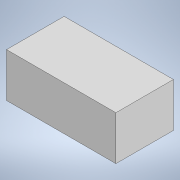
# Autodesk Inventor part: MFH-Boxdummy
Saved by Autodesk Inventor 2020 (Build 240168000, 168)
## iProperties
Created: 2020-06-04
Part Number: MFH-Boxdummy
Material: Generisch
Document SubType Name: Modeling
Designer: Chris
Density: 1 g/cm^3
Appearance: Vorgabe
Author: Chris
Autodesk Inventor part; units mm, degrees
ref_plane "YZ Plane" through (0, 0, 0) normal (1, 0, 0) x (0, 1, 0)
ref_plane "XZ Plane" through (0, 0, 0) normal (0, 1, 0) x (-1, 0, 0)
ref_plane "XY Plane" through (0, 0, 0) normal (0, 0, 1) x (1, 0, 0)
sketch "Skizze1" plane through (0, 0, 0) normal (0, 1, 0) x (-1, 0, 0)
  line L0 (0, 0) -> (570, 0)
  line L1 (570, 0) -> (570, -300)
  line L2 (570, -300) -> (0, -300)
  line L3 (0, -300) -> (0, 0)
  dimension "d0" = 570
  dimension "d1" = 300
  constraints: 8 end point, 2 parallel, 1 horizontal, 1 perpendicular
  measures "d0" distance of L1.end L2.end
  measures "d1" distance of L0.end L1.end
extrude "Extrusion1" add sketch "Skizze1" along normal blind 230
